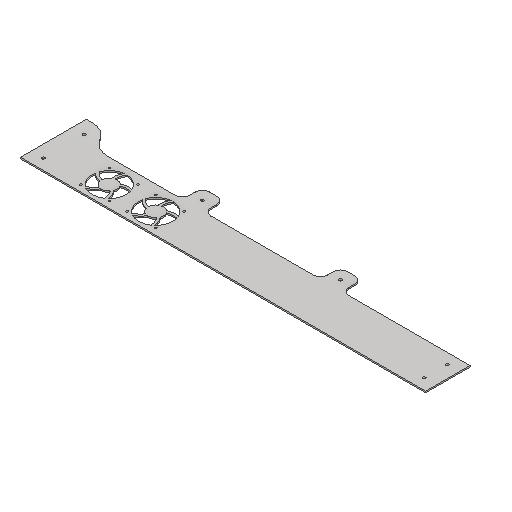
# Autodesk Inventor part: LC_ALU_2mm_Left_Plate
Saved by Autodesk Inventor 2026.1 (Build 301233000, 233)
## iProperties
Created: 2016-06-26
Part Number: LC_ALU_2mm_Left_Plate
Material: Ogólny
Document SubType Name: Modeling
Designer: Andrzej
Density: 1 g/cm^3
Appearance: Obrobione — aluminium
Mass: 73.9703 g
Surface Area: 768.735 cm^2
Volume: 73.9703 cm^3
Author: Andrzej
Autodesk Inventor part; units mm, degrees
ref_plane "YZ Plane" through (0, 0, 0) normal (1, 0, 0) x (0, 1, 0)
ref_plane "XZ Plane" through (0, 0, 0) normal (0, 1, 0) x (-1, 0, 0)
ref_plane "XY Plane" through (0, 0, 0) normal (0, 0, 1) x (1, 0, 0)
sketch "Szkic1" plane through (0, 0, 0) normal (0, 0, 1) x (1, 0, 0)
  line L0 (-98.62, 58.242) -> (467.38, 58.242)
  line L1 (467.38, 58.242) -> (467.38, -3.758)
  line L2 (467.38, -3.758) -> (-98.62, -3.758)
  line L3 (-98.62, -3.758) -> (-98.62, 58.242)
  line L4 (65.48, 58.242) -> (95.48, 58.242)
  line L5 (95.48, 58.242) -> (95.48, 86.242)
  line L6 (95.48, 86.242) -> (65.48, 86.242)
  line L7 (65.48, 86.242) -> (65.48, 58.242)
  line L8 (258.28, 58.242) -> (288.28, 58.242)
  line L9 (288.28, 58.242) -> (288.28, 86.242)
  line L10 (288.28, 86.242) -> (258.28, 86.242)
  line L11 (258.28, 86.242) -> (258.28, 58.242)
  line L12 (-98.62, 58.242) -> (-98.62, 88.242)
  line L13 (-98.62, 88.242) -> (-68.62, 88.242)
  line L14 (-68.62, 88.242) -> (-68.62, 58.242)
  line L15 (-28.62, 50.242) -> (21.38, 50.242)
  line L16 (21.38, 50.242) -> (21.38, 0.242)
  line L17 (21.38, 0.242) -> (-28.62, 0.242)
  line L18 (-28.62, 0.242) -> (-28.62, 50.242)
  circle A0 centre (-23.62, 45.242) radius 1.5
  circle A1 centre (16.38, 45.242) radius 1.5
  circle A2 centre (-23.62, 5.242) radius 1.5
  circle A3 centre (16.38, 5.242) radius 1.5
  circle A4 centre (-3.62, 25.242) radius 24
  circle A5 centre (-3.62, 25.242) radius 11
  arc A6 (9.6779, 5.2628) -> (4.7367, 18.0889) centre (-10.3192, 4.9238) ccw
  arc A7 (12.5064, 7.4673) -> (6.6011, 21.1764) centre (-7.4877, 6.9811) ccw
  arc A8 (19.4906, 31.7151) -> (5.7653, 30.9792) centre (13.6335, 12.592) ccw
  arc A9 (18.2681, 35.0864) -> (3.4051, 33.7065) centre (12.552, 15.9207) ccw
  arc A10 (-2.6348, 49.2217) -> (-6.1762, 35.9408) centre (13.7425, 37.742) ccw
  arc A11 (-6.2188, 49.1008) -> (-9.4993, 34.5389) centre (10.2425, 37.742) ccw
  arc A12 (-26.1217, 33.5891) -> (-14.5851, 26.117) centre (-10.1429, 45.6174) ccw
  arc A13 (-27.1142, 30.1431) -> (-14.2787, 22.5233) centre (-11.2244, 42.2887) ccw
  arc A14 (-18.512, 6.421) -> (-7.8406, 15.0839) centre (-25.0139, 25.3347) ccw
  arc A15 (-15.5414, 4.4122) -> (-4.3281, 14.2648) centre (-22.1823, 23.2774) ccw
  line L19 (36.38, 50.242) -> (86.38, 50.242)
  line L20 (86.38, 50.242) -> (86.38, 0.242)
  line L21 (86.38, 0.242) -> (36.38, 0.242)
  line L22 (36.38, 0.242) -> (36.38, 50.242)
  circle A16 centre (41.38, 45.242) radius 1.5
  circle A17 centre (81.38, 45.242) radius 1.5
  circle A18 centre (41.38, 5.242) radius 1.5
  circle A19 centre (81.38, 5.242) radius 1.5
  circle A20 centre (61.38, 25.242) radius 24
  circle A21 centre (61.38, 25.242) radius 11
  arc A22 (74.6779, 5.2628) -> (69.7367, 18.0889) centre (54.6808, 4.9238) ccw
  arc A23 (77.5064, 7.4673) -> (71.6011, 21.1764) centre (57.5123, 6.9811) ccw
  arc A24 (84.4906, 31.7151) -> (70.7653, 30.9792) centre (78.6335, 12.592) ccw
  arc A25 (83.2681, 35.0864) -> (68.4051, 33.7065) centre (77.552, 15.9207) ccw
  arc A26 (62.3652, 49.2217) -> (58.8238, 35.9408) centre (78.7425, 37.742) ccw
  arc A27 (58.7812, 49.1008) -> (55.5007, 34.5389) centre (75.2425, 37.742) ccw
  arc A28 (38.8783, 33.5891) -> (50.4149, 26.117) centre (54.8571, 45.6174) ccw
  arc A29 (37.8858, 30.1431) -> (50.7213, 22.5233) centre (53.7756, 42.2887) ccw
  arc A30 (46.488, 6.421) -> (57.1594, 15.0839) centre (39.9861, 25.3347) ccw
  arc A31 (49.4586, 4.4122) -> (60.6719, 14.2648) centre (42.8177, 23.2774) ccw
  point P0 (0, 0)
  point P1 (80.48, 71.242)
  point P2 (273.28, 71.242)
  point P3 (-81.62, 68.242)
  point P4 (450.38, 43.242)
  point P5 (-81.62, 11.242)
  point P6 (450.38, 11.242)
  dimension "d0" = 566
  dimension "d1" = 62
  dimension "d2" = 30
  dimension "d3" = 28
  dimension "d4" = 30
  dimension "d5" = 28
  dimension "d6" = 164.1
  dimension "d7" = 356.9
  dimension "d11" = 17
  dimension "d12" = 17
  dimension "d13" = 15
  dimension "d14" = 15
  dimension "d15" = 15
  dimension "d16" = 15
  dimension "d18" = 15
  dimension "d26" = 17
  dimension "d27" = 17
  dimension "d28" = 15
  dimension "d29" = 15
  dimension "d30" = 30
  dimension "d31" = 30
  dimension "d36" = 20
  dimension "d38" = 50
  dimension "d39" = 50
  dimension "d42" = 8
  dimension "d44" = 70
  dimension "d46" = 5
  dimension "d47" = 5
  dimension "d48" = 5
  dimension "d49" = 5
  dimension "d50" = 5
  dimension "d51" = 5
  dimension "d52" = 5
  dimension "d53" = 5
  dimension "d54" = 3
  dimension "d55" = 3
  dimension "d56" = 3
  dimension "d92" = 25
  dimension "d98" = 25
  dimension "d99" = 50
  dimension "d100" = 50
  dimension "d101" = 5
  dimension "d102" = 5
  dimension "d103" = 5
  dimension "d104" = 5
  dimension "d105" = 5
  dimension "d106" = 5
  dimension "d107" = 5
  dimension "d108" = 5
  dimension "d109" = 3
  dimension "d110" = 3
  dimension "d111" = 3
  dimension "d112" = 25
  dimension "d113" = 25
  dimension "d114" = 15
  dimension "d115" = 8
  constraints: 46 end point, 40 point on circle, 28 centre point, 12 coincident, 10 parallel, 7 perpendicular, 5 horizontal, 3 point on line, 1 vertical, 48 other
  measures "d0" distance of L1.end L2.end
  measures "d1" distance of L2.end L0.start
  measures "d2" distance of L6.end L5.end
  measures "d3" distance of L5.end L4.end
  measures "d4" distance of L10.end L9.end
  measures "d5" distance of L9.end L8.end
  measures "d6" distance between parallel lines of L3 L7
  measures "d7" distance between parallel lines of L3 L11
  measures "d11" distance from line of L3 point (-81.62, 68.242)
  measures "d12" distance from line of L1 point (450.38, 43.242)
  measures "d13" distance from line of L6 point (80.48, 71.242)
  measures "d14" distance from line of L10 point (273.28, 71.242)
  measures "d15" distance from line of L7 point (80.48, 71.242)
  measures "d16" distance from line of L11 point (273.28, 71.242)
  measures "d18" distance from line of L0 point (450.38, 43.242)
  measures "d26" distance from line of L3 point (-81.62, 11.242)
  measures "d27" distance from line of L1 point (450.38, 11.242)
  measures "d28" distance from line of L2 point (-81.62, 11.242)
  measures "d29" distance from line of L2 point (450.38, 11.242)
  measures "d30" distance of L0.start L12.end
  measures "d31" distance of L12.end L13.end
  measures "d36" distance from line of L13 point (-81.62, 68.242)
  measures "d38" distance of L16.end L17.end
  measures "d39" distance of L15.end L16.end
  measures "d42" distance between parallel lines of L0 L15
  measures "d44" distance between parallel lines of L3 L18
  measures "d46" distance from line of L18 point (-23.62, 45.242)
  measures "d47" distance from line of L15 point (-23.62, 45.242)
  measures "d48" distance from line of L18 point (-23.62, 5.242)
  measures "d49" distance from line of L17 point (-23.62, 5.242)
  measures "d50" distance from line of L17 point (16.38, 5.242)
  measures "d51" distance from line of L16 point (16.38, 5.242)
  measures "d52" distance from line of L16 point (16.38, 45.242)
  measures "d53" distance from line of L15 point (16.38, 45.242)
  measures "d54" diameter of A0
  measures "d55" diameter of A1
  measures "d56" diameter of A2
  measures "d92" distance from line of L18 point (-3.62, 25.242)
  measures "d98" distance from line of L17 point (-3.62, 25.242)
  measures "d99" distance of L21.start L22.start
  measures "d100" distance of L20.start L21.start
  measures "d101" distance from line of L22 point (41.38, 45.242)
  measures "d102" distance from line of L19 point (41.38, 45.242)
  measures "d103" distance from line of L22 point (41.38, 5.242)
  measures "d104" distance from line of L21 point (41.38, 5.242)
  measures "d105" distance from line of L21 point (81.38, 5.242)
  measures "d106" distance from line of L20 point (81.38, 5.242)
  measures "d107" distance from line of L20 point (81.38, 45.242)
  measures "d108" distance from line of L19 point (81.38, 45.242)
  measures "d109" diameter of A16
  measures "d110" diameter of A17
  measures "d111" diameter of A18
  measures "d112" distance from line of L22 point (61.38, 25.242)
  measures "d113" distance from line of L21 point (61.38, 25.242)
  measures "d114" distance between parallel lines of L16 L22
  measures "d115" distance between parallel lines of L0 L19
extrude "Wyciągnięcie proste1" add sketch "Szkic1" along normal blind 2 contours L12 L13 L14 L0 | L0 L1 L2 L3 | L7 L6 L5 L0 | L11 L10 L9 L0 | L15 L16 L17 L18 | A0 | A1 | A2 | A3 | A4 A7 A5 A8 | A8 A5 A9 A4 | A4 A6 A5 A7 | A9 A5 A10 A4 | A5 | A4 A15 A5 A6 | A10 A5 A11 A4 | A4 A14 A5 A15 | A11 A5 A12 A4 | A4 A13 A5 A14 | A12 A5 A13 A4 | L19 L20 L21 L22 | A16 | A17 | A18 | A19 | A20 A23 A21 A24 | A24 A21 A25 A20 | A20 A22 A21 A23 | A25 A21 A26 A20 | A21 | A20 A31 A21 A22 | A26 A21 A27 A20 | A20 A30 A21 A31 | A27 A21 A28 A20 | A20 A29 A21 A30 | A28 A21 A29 A20
fillet "Zaokrąglenie1" radius 10 8 edges at (95.48, 86.242, 1) (95.48, 58.242, 1) (65.48, 58.242, 1) (65.48, 86.242, 1) (258.28, 58.242, 1) (258.28, 86.242, 1) (288.28, 86.242, 1) (288.28, 58.242, 1)
hole "Otwór1" at (80.48, 71.242, 0) at (273.28, 71.242, 0) at (-81.62, 68.242, 0) at (450.38, 43.242, 0) at (-81.62, 11.242, 0) at (450.38, 11.242, 0) direction (0, 0, 1) diameter 4 end through all
fillet "Zaokrąglenie3" radius 30 2 edges at (-68.62, 58.242, 1) (-68.62, 88.242, 1)
extrude "Wyciągnięcie proste3" cut sketch "Szkic1" along normal through all contours A0 | A1 | A2 | A3 | A4 A7 A5 A8 | A9 A5 A10 A4 | A4 A15 A5 A6 | A11 A5 A12 A4 | A4 A13 A5 A14 | A16 | A17 | A18 | A19 | A20 A23 A21 A24 | A25 A21 A26 A20 | A20 A31 A21 A22 | A27 A21 A28 A20 | A20 A29 A21 A30
equation "\"d12\" = d11"
equation "\"d15\" = 0.5 * d2"
equation "\"d16\" = 0.5 * d4"
equation "\"d18\" = d17"
equation "\"d28\" = d17"
equation "\"d29\" = d18"
equation "\"d46\" = d47"
equation "\"d48\" = d47"
equation "\"d49\" = d46"
equation "\"d50\" = d46"
equation "\"d51\" = d46"
equation "\"d52\" = d46"
equation "\"d53\" = d46"
equation "\"d17\" = 15"
